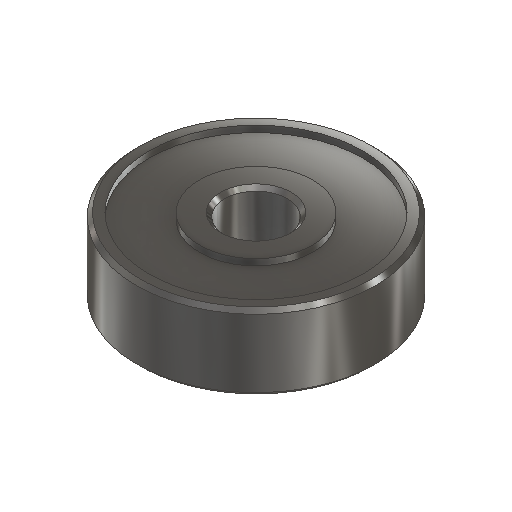
# Autodesk Inventor part: COTS_GENERIC_Bearing_19x5x6
Saved by Autodesk Inventor 2026.1 (Build 301233000, 233)
## iProperties
Created: 2017-05-27
Part Number: COTS_GENERIC_Bearing_19x5x6
Material: Ogólny
Document SubType Name: Modeling
Designer: Andrzej
Density: 1 g/cm^3
Appearance: Stal - polerowana
Mass: 1.41321 g
Surface Area: 10.3536 cm^2
Volume: 1.41321 cm^3
Author: Andrzej
Autodesk Inventor part; units mm, degrees
ref_plane "YZ Plane" through (0, 0, 0) normal (1, 0, 0) x (0, 1, 0)
ref_plane "XZ Plane" through (0, 0, 0) normal (0, 1, 0) x (-1, 0, 0)
ref_plane "XY Plane" through (0, 0, 0) normal (0, 0, 1) x (1, 0, 0)
sketch "Szkic1" plane through (0, 0, 0) normal (0, 0, 1) x (1, 0, 0)
  circle A0 centre (0, 0) radius 2.5
  circle A1 centre (0, 0) radius 9.5
  dimension "d0" = 5
  dimension "d1" = 19
  constraints: 2 centre point, 2 coincident
  measures "d0" diameter of A0
  measures "d1" diameter of A1
extrude "Wyciągnięcie proste1" add sketch "Szkic1" along normal blind 6
chamfer "Faza1" distance 0.3 angle 45 4 edges at (-9.5, 0, 6) (-2.5, 0, 6) (-9.5, 0, 0) (-2.5, 0, 0)
sketch "Szkic2" plane through (0, 0, 0) normal (0, 0, -1) x (-1, 0, 0)
  circle A0 centre (0, 0) radius 9.2 projected
  circle A1 centre (0, 0) radius 2.8 projected
  circle A2 centre (0, 0) radius 9.5 projected
  circle A3 centre (0, 0) radius 2.5 projected
  circle A4 centre (0, 0) radius 4.5
  circle A5 centre (0, 0) radius 8.5
  dimension "d7" = 2
  dimension "d8" = 1
  constraints: 2 centre point
  measures "d7" radial gap between concentric circles of A3 A4
  measures "d8" radial gap between concentric circles of A2 A5
extrude "Wyciągnięcie proste2" cut sketch "Szkic2" against normal blind 0.5 contours A5
sketch "Szkic3" plane through (0, 0, 6) normal (0, 0, 1) x (1, 0, 0)
  circle A0 centre (0, 0) radius 8.5 projected
  circle A1 centre (0, 0) radius 4.5 projected
extrude "Wyciągnięcie proste3" cut sketch "Szkic3" against normal blind 0.5
